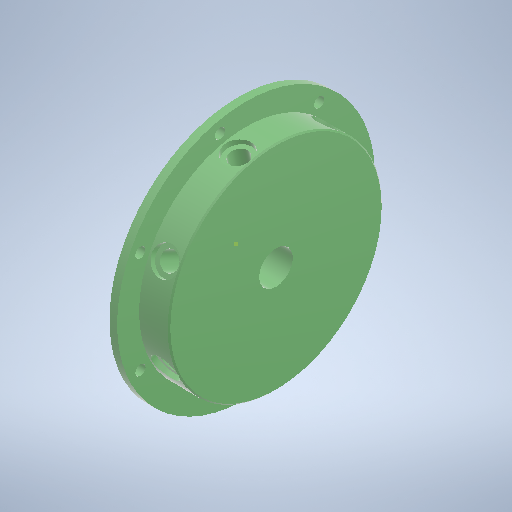
# Autodesk Inventor part: Decke_grün
Saved by Autodesk Inventor 2025 (Build 290162010, 162A)
## iProperties
Created: 2024-03-08
Part Number: Decke_grün
Material: Generisch
Document SubType Name: Modeling
Designer: ffogue
Density: 1 g/cm^3
Appearance: Glatt - Waldgrün
Author: ffogue
Autodesk Inventor part; units mm, degrees
note: some values were not read from the file. Chosen so that the rebuilt part matches the saved one: direction of "Bohrung1".
ref_plane "YZ Plane" through (0, 0, 0) normal (1, 0, 0) x (0, 1, 0)
ref_plane "XY Plane" through (0, 0, 0) normal (0, 0, 1) x (1, 0, 0)
sketch "Skizze1" plane through (0, 0, 0) normal (0, 0, 1) x (1, 0, 0)
  line L0 (0, 0) -> (15.5, 0)
  line L1 (0, 0) -> (0, 42.25)
  line L2 (0, 42.25) -> (0.9, 42.25)
  line L3 (0.9, 42.25) -> (0.9, 50)
  line L4 (0.9, 50) -> (3.9, 50)
  line L5 (3.9, 50) -> (3.9, 41.5)
  line L6 (3.9, 41.5) -> (15.5, 41.5)
  line L7 (15.5, 41.5) -> (15.5, 0)
  dimension "d0" = 15.5
  dimension "d1" = 0.9
  dimension "d2" = 3
  dimension "d3" = 100
  dimension "d4" = 84.5
  dimension "d5" = 83
  constraints: 16 end point, 6 perpendicular, 1 coincident, 1 horizontal, 1 vertical
  measures "d0" distance of L0.start L0.end
  measures "d1" distance between parallel lines of L3 L1
  measures "d2" distance between parallel lines of L5 L3
  measures "d3" diameter of L4 L0
  measures "d4" diameter of L2 L0
  measures "d5" diameter of L6 L0
revolve "Umdrehung1" add sketch "Skizze1" angle 360 about axis through (0, 0, 0) along (1, 0, 0)
sketch "Skizze2" plane through (3.9, 0, 0) normal (1, 0, 0) x (0, 0, -1)
  circle A0 centre (0, 0) radius 45.5 construction
  line L0 (0, -70) -> (0, 70) construction
  point P0 (0, 45.5)
  dimension "d7" = 91
  constraints: 1 coincident, 1 point on line, 1 vertical alignment, 2 other
hole "Bohrung1" at (3.9, 45.5, 0) direction (-1, 0, 0) diameter 4 depth 3
pattern_circular "Runde Anordnung1" count 7 over 360 about axis through (2.4, 0, 0) along (1, 0, 0) of "Bohrung1"
sketch "Skizze3" plane through (15.5, 0, 0) normal (1, 0, 0) x (0, 0, -1)
  circle A0 centre (0, 0) radius 6.5
  dimension "d18" = 13
  constraints: 1 centre point, 1 coincident
  measures "d18" diameter of A0
extrude "Extrusion1" cut sketch "Skizze3" against normal up to surface (15.5 mm away)
ref_plane "Arbeitsebene2" through (0, 41.5, 0) normal (0, 1, 0) x (-1, 0, 0)
sketch "Skizze5" plane through (0, 41.5, 0) normal (0, 1, 0) x (-1, 0, 0)
  line L0 (-3.9, 50) -> (-3.9, -50) projected
  point P0 (0, 0)
  point P1 (-9.9, 0)
  dimension "d23" = 6
  constraints: 1 horizontal alignment
  measures "d23" distance from line of L0 point (-9.9, 0)
hole "Bohrung2" at (9.9, 41.5, 0) direction (0, -1, 0) diameter 7 depth 5 counterbore diameter 10.5 counterbore depth 2
sketch "Skizze6" plane through (0, 0, 0) normal (-1, 0, 0) x (0, 0, 1)
  point P0 (0, 0)
sketch "Skizze7" plane through (9.9, 39.5, 0) normal (0, 1, 0) x (1, 0, 0)
  circle A0 centre (0, 0) radius 3.5 projected
  circle A1 centre (0, 0) radius 4
  point P0 (-9.9, 0)
  dimension "d31" = 8
  constraints: 1 centre point, 1 coincident
  measures "d31" diameter of A1
extrude "Extrusion2" cut sketch "Skizze7" against normal blind 22 contours A0
sketch "Skizze8" plane through (0, 0, 0) normal (-1, 0, 0) x (0, 0, 1)
  circle A0 centre (0, 17) radius 4.5
  point P0 (0, 0)
  dimension "d34" = 17
  dimension "d35" = 9
  constraints: 1 centre point, 1 vertical alignment
  measures "d34" distance of A0.centre point (0, 0)
  measures "d35" diameter of A0
extrude "Extrusion3" cut sketch "Skizze8" against normal blind 15
pattern_circular "Runde Anordnung2" count 7 over 360 about axis through (9.7, 0, 0) along (1, 0, 0) of "Bohrung2"
pattern_circular "Runde Anordnung3" count 7 over 360 about axis through (0.45, 0, 0) along (1, 0, 0) of "Extrusion3"
pattern_circular "Runde Anordnung4" count 7 over 360 about axis through (9.7, 0, 0) along (1, 0, 0) of "Extrusion2"
chamfer "Fasen1" distance 0.5 angle 45 1 edges at (15.5, -41.5, 0)
